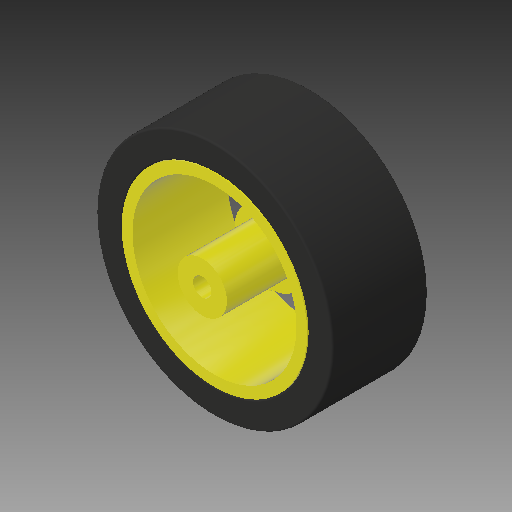
# Autodesk Inventor part: 輪胎
Saved by Autodesk Inventor 2017 (Build 210142000, 142)
## iProperties
Created: 2019-10-03
Part Number: 輪胎
Material: Generic
Document SubType Name: Modeling
Designer: User
Density: 1 g/cm^3
Appearance: Default
Mass: 52.6859 g
Surface Area: 170.593 cm^2
Volume: 52.6859 cm^3
Author: User
Autodesk Inventor part; units mm, degrees
ref_plane "YZ Plane" through (0, 0, 0) normal (1, 0, 0) x (0, 1, 0)
ref_plane "Work Plane1" through (0, 0, 13.3) normal (0, 0, 1) x (1, 0, 0)
sketch "Sketch2" plane through (0, 0, 13.3) normal (0, 0, 1) x (1, 0, 0)
  circle A0 centre (0, 0) radius 25.9
  circle A1 centre (0, 0) radius 22.9
  dimension "d5" = 45.8
  constraints: 2 centre point, 2 coincident
  measures "d5" diameter of A1
extrude "Extrusion2" add sketch "Sketch2" against normal blind 26.6
sketch "Sketch3" plane through (0, 0, 0) normal (0, 1, 0) x (-1, 0, 0)
  line L0 (25.9, 12.8) -> (25.9, 12.3)
  line L1 (33, 12.3) -> (33, 12.8)
  line L2 (32.5, 13.3) -> (26.4, 13.3)
  line L3 (33, 12.8) -> (33, 0)
  line L4 (25.9, 12.3) -> (25.9, 0)
  line L5 (25.9, 13.3) -> (25.9, -13.3) projected
  arc A0 (33, 12.8) -> (32.5, 13.3) centre (32.5, 12.8) ccw
  arc A1 (26.4, 13.3) -> (25.9, 12.8) centre (26.4, 12.8) ccw
  line L6 (25.9, -12.8) -> (25.9, -12.3)
  line L7 (32.5, -13.3) -> (26.4, -13.3)
  line L8 (33, -12.8) -> (33, 0)
  line L9 (25.9, -12.3) -> (25.9, 0)
  arc A2 (32.5, -13.3) -> (33, -12.8) centre (32.5, -12.8) ccw
  arc A3 (25.9, -12.8) -> (26.4, -13.3) centre (26.4, -12.8) ccw
  line L10 (0, -18.765) -> (0, 18.765) projected
  point P0 (0, 0)
  dimension "d10" = 0.5
  constraints: 18 end point, 8 point on circle, 4 centre point, 4 tangent, 1 equal radius, 1 horizontal, 1 midpoint, 1 point on line, 1 vertical
  measures "d10" radius of A0
revolve "Revolution1" add sketch "Sketch3" angle 360 about axis through (0, 0, -10) along (0, 0, 1)
sketch "Sketch4" plane through (0, 0, -13.3) normal (0, 0, -1) x (-1, 0, 0)
  line L0 (0, 0) -> (22.9, 0) construction
  line L1 (0, 0) -> (22.9, 0) construction
  line L2 (0, 0) -> (22.9, 0) construction
  line L3 (0, 0) -> (22.9, 0) construction
  line L4 (0, 0) -> (22.9, 0) construction
  line L5 (0, 0) -> (22.9, 0) construction
  line L6 (-3.9765, 22.5521) -> (-5.1908, 13.316)
  line L7 (-20.2195, 10.7509) -> (-11.0602, 9.0516)
  arc A0 (-11.0602, 9.0516) -> (-5.1908, 13.316) centre (-10.1482, 13.9677) ccw
  arc A1 (-12.0264, -7.7218) -> (-14.2683, -0.8219) centre (-16.4201, -5.3352) ccw
  line L8 (-16.4729, -15.9077) -> (-12.0264, -7.7218)
  line L9 (-22.6771, 3.1871) -> (-14.2683, -0.8219)
  arc A2 (3.6275, -13.8239) -> (-3.6275, -13.8239) centre (0, -17.2651) ccw
  line L10 (10.0387, -20.5824) -> (3.6275, -13.8239)
  line L11 (-10.0387, -20.5824) -> (-3.6275, -13.8239)
  arc A3 (14.2683, -0.8219) -> (12.0264, -7.7218) centre (16.4201, -5.3352) ccw
  line L12 (22.6771, 3.1871) -> (14.2683, -0.8219)
  line L13 (16.4729, -15.9077) -> (12.0264, -7.7218)
  arc A4 (5.1908, 13.316) -> (11.0602, 9.0516) centre (10.1482, 13.9677) ccw
  line L14 (3.9765, 22.5521) -> (5.1908, 13.316)
  line L15 (20.2195, 10.7509) -> (11.0602, 9.0516)
  arc A5 (-20.2195, 10.7509) -> (-22.6771, 3.1871) centre (0, 0) ccw
  arc A6 (3.9765, 22.5521) -> (-3.9765, 22.5521) centre (0, 0) ccw
  arc A7 (22.6771, 3.1871) -> (20.2195, 10.7509) centre (0, 0) ccw
  arc A8 (-16.4729, -15.9077) -> (-10.0387, -20.5824) centre (0, 0) ccw
  arc A9 (10.0387, -20.5824) -> (16.4729, -15.9077) centre (0, 0) ccw
  dimension "d22" = 360
  constraints: 32 end point, 20 point on circle, 10 centre point, 6 horizontal, 2 coincident, 2 tangent, 41 other
extrude "Extrusion3" add sketch "Sketch4" against normal blind 1
sketch "Sketch7" plane through (0, 0, 0) normal (1, 0, 0) x (0, 1, 0)
  line L0 (10.7509, -13.3) -> (22.5521, -13.3) projected
  line L1 (13.316, -13.3) -> (22.5521, -13.3) projected
  line L2 (9.0516, -13.3) -> (13.316, -13.3) projected
  line L3 (10.7509, -13.3) -> (9.0516, -13.3) projected
  line L4 (-0.8219, -13.3) -> (3.1871, -13.3) projected
  line L5 (-7.7218, -13.3) -> (-0.8219, -13.3) projected
  line L6 (-15.9077, -13.3) -> (-7.7218, -13.3) projected
  line L7 (-15.9077, -13.3) -> (3.1871, -13.3) projected
  line L8 (-13.8239, -13.3) -> (-20.5824, -13.3) projected
  line L9 (-13.8239, -13.3) -> (-13.8239, -13.3) projected
  line L10 (-20.5824, -13.3) -> (-13.8239, -13.3) projected
  line L11 (-20.5824, -13.3) -> (-20.5824, -13.3) projected
  line L12 (-7.7218, -13.3) -> (-15.9077, -13.3) projected
  line L13 (-0.8219, -13.3) -> (-7.7218, -13.3) projected
  line L14 (3.1871, -13.3) -> (-0.8219, -13.3) projected
  line L15 (3.1871, -13.3) -> (-15.9077, -13.3) projected
  line L16 (9.0516, -13.3) -> (10.7509, -13.3) projected
  line L17 (13.316, -13.3) -> (9.0516, -13.3) projected
  line L18 (22.5521, -13.3) -> (13.316, -13.3) projected
  line L19 (22.5521, -13.3) -> (10.7509, -13.3) projected
  line L20 (-25.9, -13.3) -> (25.9, -13.3) projected
  line L21 (-22.9, 13.3) -> (22.9, 13.3) projected
  line L22 (10.7509, -13.3) -> (10.7509, -12.3) projected
  line L23 (10.7509, -12.3) -> (3.1871, -12.3) projected
  line L24 (3.1871, -12.3) -> (3.1871, -13.3) projected
  line L25 (-15.9077, -13.3) -> (3.1871, -13.3) projected
  line L26 (-15.9077, -13.3) -> (-15.9077, -12.3) projected
  line L27 (-15.9077, -12.3) -> (-20.5824, -12.3) projected
  line L28 (-20.5824, -12.3) -> (-20.5824, -13.3) projected
  line L29 (-20.5824, -13.3) -> (-20.5824, -13.3) projected
  line L30 (-20.5824, -13.3) -> (-20.5824, -12.3) projected
  line L31 (-20.5824, -12.3) -> (-15.9077, -12.3) projected
  line L32 (-15.9077, -12.3) -> (-15.9077, -13.3) projected
  line L33 (3.1871, -13.3) -> (-15.9077, -13.3) projected
  line L34 (3.1871, -13.3) -> (3.1871, -12.3) projected
  line L35 (3.1871, -12.3) -> (10.7509, -12.3) projected
  line L36 (10.7509, -12.3) -> (10.7509, -13.3) projected
  line L37 (22.5521, -13.3) -> (10.7509, -13.3) projected
  line L38 (22.5521, -12.3) -> (22.5521, -12.3) projected
  line L39 (10.7509, -13.3) -> (22.5521, -13.3) projected
  line L40 (-22.9, 13.3) -> (22.9, 13.3) projected
  line L41 (10.7509, -13.3) -> (10.7509, -12.3) projected
  line L42 (10.7509, -12.3) -> (3.1871, -12.3) projected
  line L43 (3.1871, -12.3) -> (3.1871, -13.3) projected
  line L44 (-15.9077, -13.3) -> (3.1871, -13.3) projected
  line L45 (-15.9077, -13.3) -> (-15.9077, -12.3) projected
  line L46 (-15.9077, -12.3) -> (-20.5824, -12.3) projected
  line L47 (-20.5824, -12.3) -> (-20.5824, -13.3) projected
  line L48 (-20.5824, -13.3) -> (-20.5824, -13.3) projected
  line L49 (-20.5824, -13.3) -> (-20.5824, -12.3) projected
  line L50 (-20.5824, -12.3) -> (-15.9077, -12.3) projected
  line L51 (-15.9077, -12.3) -> (-15.9077, -13.3) projected
  line L52 (3.1871, -13.3) -> (-15.9077, -13.3) projected
  line L53 (3.1871, -13.3) -> (3.1871, -12.3) projected
  line L54 (3.1871, -12.3) -> (10.7509, -12.3) projected
  line L55 (10.7509, -12.3) -> (10.7509, -13.3) projected
  line L56 (22.5521, -13.3) -> (10.7509, -13.3) projected
  line L57 (22.5521, -13.3) -> (22.5521, -12.3) projected
  line L58 (22.5521, -12.3) -> (22.5521, -12.3) projected
  line L59 (22.5521, -12.3) -> (22.5521, -13.3) projected
  line L60 (10.7509, -13.3) -> (22.5521, -13.3) projected
  line L61 (22.9, 13.3) -> (22.9, -12.3) projected
  line L62 (22.9, 13.3) -> (22.9, -12.3) projected
  line L63 (22.9, -11.2241) -> (22.9, -13.3)
  line L64 (22.4, -13.3) -> (21.9, -13.3)
  line L65 (22.5521, -12.3) -> (22.9, -12.3) projected
  line L66 (22.9, -12.8) -> (22.9, -12.3)
  arc A0 (22.4, -13.3) -> (22.9, -12.8) centre (22.4, -12.8) ccw
  line L67 (22.4, -13.3) -> (22.588, -13.3)
  line L68 (22.9, -12.8) -> (22.9, -13.3)
  line L69 (22.9, -13.3) -> (22.4, -13.3)
  line L70 (22.9, -12.8) -> (22.9, -13.3)
  line L71 (22.9, -13.3) -> (22.4, -13.3)
  line L72 (-25.9, -13.3) -> (25.9, -13.3) projected
  line L73 (0, -18.7443) -> (0, 18.6407) projected
  point P0 (0, 0)
  dimension "d28" = 1
  dimension "d29" = 0.5
  constraints: 16 end point, 7 point on line, 6 tangent, 3 collinear, 2 point on circle, 1 centre point, 1 horizontal, 1 vertical, 1 other
  measures "d28" distance of L63.end L64.end
  measures "d29" radius of A0
revolve "Revolution2" cut sketch "Sketch7" angle 360 about axis through (0, 0, -10) along (0, 0, 1) contours A0 L57 L0 | L57 A0 L63 L20
sketch "Sketch8" plane through (0, 0, -12.3) normal (0, 0, 1) x (1, 0, 0)
  circle A0 centre (0, 0) radius 10
  dimension "d31" = 20
  constraints: 1 centre point, 1 coincident
  measures "d31" diameter of A0
extrude "Extrusion4" add sketch "Sketch8" along normal blind 10
fillet "Fillet1" radius 0.2 15 edges at (6.8331, -17.2032, -12.3) (-6.8331, -17.2032, -12.3) (0, -12.2651, -12.3) (11.6648, -3.7901, -12.3) (18.4727, 1.1826, -12.3) (14.2496, -11.8147, -12.3) (4.5837, 17.934, -12.3) (15.6399, 9.9013, -12.3) (7.2092, 9.9227, -12.3) (-15.6399, 9.9013, -12.3) (-4.5837, 17.934, -12.3) (-7.2092, 9.9227, -12.3) (-14.2496, -11.8147, -12.3) (-18.4727, 1.1826, -12.3) (-11.6648, -3.7901, -12.3) curvature continuous yes
fillet "Fillet2" radius 0.3 5 edges at (-16.1927, -16.1927, -13.3) (22.8442, 1.5974, -13.3) (13.4603, 18.5265, -13.3) (1.9959, 22.8129, -13.3) (21.7792, 7.0765, -13.3) curvature continuous yes
sketch "Sketch9" plane through (0, 0, -13.3) normal (0, 0, -1) x (-1, 0, 0)
  circle A0 centre (0, 0) radius 10
  dimension "d36" = 20
  constraints: 1 centre point, 1 coincident
  measures "d36" diameter of A0
ref_plane "Work Plane2" through (0, 0, -8.3) normal (0, 0, -1) x (-1, 0, 0)
sketch "Sketch10" plane through (0, 0, -8.3) normal (0, 0, -1) x (-1, 0, 0)
  circle A0 centre (0, 0) radius 7.5
  dimension "d38" = 15
  constraints: 1 centre point, 1 coincident
  measures "d38" diameter of A0
loft "Loft1" cut profiles "Sketch10", "Sketch9"
fillet "Fillet3" radius 0.5 2 edges at (10, 0, -13.3) (7.5, 0, -8.3)
sketch "Sketch11" plane through (0, 0, -8.3) normal (0, 0, -1) x (-1, 0, 0)
  circle A0 centre (0, 0) radius 3.75
  circle A1 centre (0, 5.5) radius 0.5
  circle A2 centre (-5.2308, 1.6996) radius 0.5
  circle A3 centre (-3.2328, -4.4496) radius 0.5
  circle A4 centre (3.2328, -4.4496) radius 0.5
  circle A5 centre (5.2308, 1.6996) radius 0.5
  dimension "d44" = 7.5
  dimension "d45" = 1
  dimension "d48" = 360
  constraints: 6 centre point, 1 coincident, 11 other
  measures "d44" diameter of A0
  measures "d45" diameter of A1
extrude "Extrusion5" add sketch "Sketch11" along normal blind 2
fillet "Fillet4" radius 0.5 6 edges at (3.75, 0, -10.3) (5.7308, 1.6996, -10.3) (0.5, 5.5, -10.3) (-4.7308, 1.6996, -10.3) (-2.7328, -4.4496, -10.3) (3.7328, -4.4496, -10.3)
sketch "Sketch12" plane through (0, 0, -2.3) normal (0, 0, 1) x (1, 0, 0)
  circle A0 centre (0, 0) radius 6.9
  dimension "d53" = 13.8
  constraints: 1 centre point, 1 coincident
  measures "d53" diameter of A0
extrude "Extrusion6" add sketch "Sketch12" along normal blind 19
sketch "Sketch13" plane through (0, 0, 16.7) normal (0, 0, 1) x (1, 0, 0)
  circle A0 centre (0, 0) radius 2.55
  dimension "d56" = 5.1
  constraints: 1 centre point, 1 coincident
  measures "d56" diameter of A0
extrude "Extrusion7" cut sketch "Sketch13" against normal blind 15
body "Solid1"
